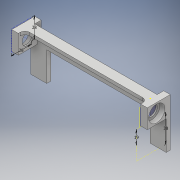
# Autodesk Inventor part: rearAxelHolder 9-19
Saved by Autodesk Inventor 2018 (Build 220112000, 112)
## iProperties
Created: 2019-09-19
Part Number: rearAxelHolder 9-19
Material: Generic
Document SubType Name: Modeling
Designer: Aditya Kendre
Density: 1 g/cm^3
Appearance: Default
Author: Aditya Kendre
Autodesk Inventor part; units mm, degrees
ref_plane "YZ Plane" through (0, 0, 0) normal (1, 0, 0) x (0, 1, 0)
ref_plane "XZ Plane" through (0, 0, 0) normal (0, 1, 0) x (-1, 0, 0)
ref_plane "XY Plane" through (0, 0, 0) normal (0, 0, 1) x (1, 0, 0)
sketch "Sketch1" plane through (0, 0, 0) normal (1, 0, 0) x (0, 1, 0)
  circle A0 centre (0, 0) radius 11.25
  line L0 (-11.25, 11.25) -> (11.25, 11.25) construction
  line L1 (11.25, 11.25) -> (11.25, -11.25) construction
  line L2 (11.25, -11.25) -> (-11.25, -11.25) construction
  line L3 (-11.25, -11.25) -> (-11.25, 11.25) construction
  line L4 (-11.25, 11.25) -> (11.25, -11.25) construction
  line L5 (11.25, 11.25) -> (-11.25, -11.25) construction
  line L6 (11.25, 11.25) -> (14.25, 11.25) construction
  line L7 (14.25, 11.25) -> (14.25, -11.25) construction
  line L8 (14.25, -11.25) -> (11.25, -11.25) construction
  line L9 (11.25, -11.25) -> (11.25, 11.25) construction
  line L10 (14.25, -11.25) -> (-11.25, -11.25) construction
  line L11 (-11.25, -11.25) -> (-11.25, -14.25) construction
  line L12 (-11.25, -14.25) -> (14.25, -14.25) construction
  line L13 (14.25, -14.25) -> (14.25, -11.25) construction
  line L14 (-13, 13) -> (13, 13)
  line L15 (13, 13) -> (13, -13)
  line L16 (13, -13) -> (-13, -13)
  line L17 (-13, -13) -> (-13, 13)
  line L18 (-13, 13) -> (13, -13) construction
  line L19 (13, 13) -> (-13, -13) construction
  dimension "d0" = 22.5
  dimension "d1" = 3
  dimension "d2" = 3
  dimension "d3" = 26
  dimension "d4" = 26
  constraints: 40 end point, 8 parallel, 4 horizontal, 4 midpoint, 4 perpendicular, 1 centre point, 1 coincident
  measures "d0" diameter of A0
  measures "d1" distance of L7.end L8.end
  measures "d2" distance of L11.end L10.end
  measures "d3" distance of L15.end L16.end
  measures "d4" distance of L14.end L15.end
extrude "Extrusion1" add sketch "Sketch1" along normal blind 9
sketch "Sketch2" plane through (0, 0, 0) normal (-1, 0, 0) x (0, 0, 1)
  circle A0 centre (0, 0) radius 7.75
  circle A1 centre (0, 0) radius 11.25
  dimension "d7" = 15.5
  constraints: 2 centre point, 2 coincident
  measures "d7" diameter of A0
extrude "Extrusion2" add sketch "Sketch2" against normal blind 2
sketch "Sketch3" plane through (0, 0, 0) normal (-1, 0, 0) x (0, 0, 1)
  line L0 (13, 13) -> (-13, 13) projected
  line L1 (13, 13) -> (8.75, 13)
  line L2 (8.75, 13) -> (8.75, -13)
  line L3 (8.75, -13) -> (13, -13)
  line L4 (13, -13) -> (13, 13)
  point P0 (0, 0)
  dimension "d10" = 4.25
  dimension "d11" = 26
  constraints: 8 end point, 2 parallel, 1 horizontal, 1 perpendicular
  measures "d10" distance of L3.end L2.end
  measures "d11" distance of L2.end L1.end
extrude "Extrusion3" add sketch "Sketch3" along normal blind 168
sketch "Sketch4" plane through (-168, 0, 0) normal (-1, 0, 0) x (0, 0, 1)
  line L0 (13, 13) -> (13, -13) projected
  line L1 (-13, -13) -> (-13, 13) projected
  line L2 (13, -13) -> (-13, -13)
  line L3 (-13, -13) -> (-13, 13)
  line L4 (-13, 13) -> (13, 13)
  line L5 (13, 13) -> (13, -13)
  circle A0 centre (0, 0) radius 7.75
  circle A1 centre (0, 0) radius 11.25
  constraints: 8 end point, 2 centre point, 2 coincident, 2 parallel, 1 horizontal, 1 perpendicular
extrude "Extrusion4" add sketch "Sketch4" along normal blind 9 contours L0 L2 L1 L4
sketch "Sketch5" plane through (-168, 0, 0) normal (1, 0, 0) x (0, 0, -1)
  circle A0 centre (0, 0) radius 7.75
  circle A1 centre (0, 0) radius 11.25
  constraints: 2 centre point, 2 coincident
extrude "Extrusion5" add sketch "Sketch5" against normal blind 2
sketch "Sketch6" plane through (0, 13, -13) normal (0, 1, 0) x (1, 0, 0)
  line L0 (9, -26) -> (9, 0) projected
  line L1 (-177, -26) -> (-177, 0) projected
  line L2 (9, 0) -> (-177, 0)
  line L3 (-177, 0) -> (-177, -26)
  line L4 (-177, -26) -> (9, -26)
  line L5 (9, -26) -> (9, 0)
  point P0 (0, -13)
  constraints: 8 end point, 2 parallel, 1 horizontal, 1 perpendicular
extrude "Extrusion6" add sketch "Sketch6" along normal blind 5.5
ref_plane "Work Plane1" through (0, 0, 0) normal (-1, 0, 0) x (0, 0, 1)
sketch "Sketch7" plane through (0, 0, 0) normal (-1, 0, 0) x (0, 0, 1)
  line L0 (13, -13) -> (13, 18.5) projected
  line L1 (13, 18.5) -> (3.75, 18.5)
  line L2 (3.75, 18.5) -> (3.75, 9.5)
  line L3 (3.75, 9.5) -> (13, 9.5)
  line L4 (13, 9.5) -> (13, 18.5)
  point P0 (0, 0)
  dimension "d21" = 9.25
  dimension "d22" = 9
  constraints: 8 end point, 2 parallel, 1 horizontal, 1 perpendicular
  measures "d21" distance of L3.end L2.end
  measures "d22" distance of L2.end L1.end
extrude "Extrusion7" cut sketch "Sketch7" along normal blind 168
sketch "Sketch8" plane through (0, 0, 0) normal (-1, 0, 0) x (0, 0, 1)
  point P0 (0, 0)
sketch "Sketch9" plane through (-177, -13, 13) normal (0, 0, 1) x (1, 0, 0)
  point P0 (177, 13)
sketch "Sketch10" plane through (-177, -13, 13) normal (0, 0, 1) x (1, 0, 0)
  line L0 (0, 0) -> (0, 31.5) construction
  line L1 (9, 0) -> (0, 0) construction
  line L2 (0, 31.5) -> (9, 31.5) construction
  line L3 (9, 31.5) -> (9, 0) construction
  line L4 (9, 0) -> (0, 0) construction
  line L5 (0, 0) -> (0, 31.5) construction
  line L6 (186, 31.5) -> (0, 31.5) construction
  line L7 (0, 0) -> (186, 0) construction
  line L8 (186, 31.5) -> (177, 31.5) construction
  line L9 (177, 31.5) -> (177, 0) construction
  line L10 (177, 0) -> (186, 0) construction
  line L11 (186, 0) -> (186, 31.5) construction
  line L12 (9, 22.5) -> (9, 0) projected
  line L13 (177, 0) -> (177, 22.5) projected
  line L14 (9, 0) -> (177, 0)
  line L15 (177, 0) -> (177, 9)
  line L16 (177, 9) -> (9, 9)
  line L17 (9, 9) -> (9, 0)
  point P0 (177, 13)
  dimension "d25" = 9
  constraints: 24 end point, 6 parallel, 3 horizontal, 3 perpendicular, 2 point on line
  measures "d25" distance of L15.end L14.end
extrude "Extrusion8" cut sketch "Sketch10" against normal blind 5
fillet "Fillet1" radius 6.5 2 edges at (0, -4, 10.875) (-168, -4, 10.875)
sketch "Sketch11" plane through (9, -13, -13) normal (0, 0, -1) x (-1, 0, 0)
  point P0 (9, 13)
sketch "Sketch12" plane through (9, -13, -13) normal (0, 0, -1) x (-1, 0, 0)
  line L0 (0, 31.5) -> (186, 31.5) construction
  line L1 (9, 26) -> (177, 26) construction
  line L2 (0, 31.5) -> (22, 31.5) construction
  line L3 (22, 31.5) -> (22, 26) construction
  line L4 (22, 26) -> (0, 26) construction
  line L5 (0, 26) -> (0, 31.5) construction
  line L6 (17.1, 27.15) -> (4.9, 27.15) construction
  line L7 (4.9, 27.15) -> (4.9, 30.35) construction
  line L8 (4.9, 30.35) -> (17.1, 30.35) construction
  line L9 (17.1, 30.35) -> (17.1, 27.15) construction
  line L10 (17.1, 27.15) -> (4.9, 30.35) construction
  line L11 (4.9, 27.15) -> (17.1, 30.35) construction
  line L12 (17.1, 27.15) -> (4.9, 27.15)
  line L13 (4.9, 27.15) -> (4.9, 30.35)
  line L14 (4.9, 30.35) -> (17.1, 30.35)
  line L15 (17.1, 30.35) -> (17.1, 27.15)
  line L16 (17.1, 27.15) -> (4.9, 30.35) construction
  line L17 (4.9, 27.15) -> (17.1, 30.35) construction
  line L18 (186, 0) -> (186, 31.5) construction
  line L19 (186, 31.5) -> (164, 31.5) construction
  line L20 (164, 31.5) -> (164, 26) construction
  line L21 (164, 26) -> (186, 26) construction
  line L22 (186, 26) -> (186, 31.5) construction
  line L23 (181.1, 27.15) -> (168.9, 27.15)
  line L24 (168.9, 27.15) -> (168.9, 30.35)
  line L25 (168.9, 30.35) -> (181.1, 30.35)
  line L26 (181.1, 30.35) -> (181.1, 27.15)
  line L27 (181.1, 27.15) -> (168.9, 30.35) construction
  line L28 (168.9, 27.15) -> (181.1, 30.35) construction
  line L29 (22, 26) -> (0, 26)
  line L30 (0, 26) -> (0, 31.5)
  line L31 (0, 31.5) -> (22, 31.5)
  line L32 (22, 31.5) -> (22, 26)
  line L33 (164, 26) -> (186, 26)
  line L34 (186, 26) -> (186, 31.5)
  line L35 (186, 31.5) -> (164, 31.5)
  line L36 (164, 31.5) -> (164, 26)
  point P0 (9, 13)
  point P1 (11, 28.75)
  point P2 (175, 28.75)
  dimension "d29" = 22
  dimension "d30" = 12.2
  dimension "d31" = 3.2
  dimension "d32" = 22
  dimension "d33" = 12.2
  dimension "d34" = 3.2
  constraints: 68 end point, 14 parallel, 7 horizontal, 7 perpendicular, 6 midpoint, 2 point on line
  measures "d29" distance of L3.end L4.end
  measures "d30" distance of L7.end L8.end
  measures "d31" distance of L6.end L7.end
  measures "d32" distance of L21.end L20.end
  measures "d33" distance of L24.end L25.end
  measures "d34" distance of L23.end L24.end
extrude "Extrusion9" add sketch "Sketch12" along normal blind 40
sketch "Sketch13" plane through (4.1, 17.35, -13) normal (0, 0, -1) x (-1, 0, 0)
  line L0 (0, 0) -> (12.2, 0) projected
  line L1 (0, -3.2) -> (12.2, -3.2) projected
  line L2 (0, 0) -> (12.2, 0)
  line L3 (12.2, 0) -> (12.2, -3.2)
  line L4 (12.2, -3.2) -> (0, -3.2)
  line L5 (0, -3.2) -> (0, 0)
  line L6 (176.2, 0) -> (164, 0) projected
  line L7 (164, -3.2) -> (176.2, -3.2) projected
  line L8 (164, 0) -> (176.2, 0)
  line L9 (176.2, 0) -> (176.2, -3.2)
  line L10 (176.2, -3.2) -> (164, -3.2)
  line L11 (164, -3.2) -> (164, 0)
  point P0 (4.1, -17.35)
  constraints: 16 end point, 4 parallel, 2 horizontal, 2 perpendicular
extrude "Extrusion10" cut sketch "Sketch13" against normal blind 15
sketch "Sketch14" plane through (-177, 0, 0) normal (-1, 0, 0) x (0, 0, 1)
  line L0 (14, -14) -> (-14, -14) construction
  line L1 (-14, -14) -> (-14, 14) construction
  line L2 (-14, 14) -> (14, 14) construction
  line L3 (14, 14) -> (14, -14) construction
  line L4 (14, -14) -> (-14, 14) construction
  line L5 (-14, -14) -> (14, 14) construction
  point P0 (0, 0)
  dimension "d39" = 28
  dimension "d40" = 28
  constraints: 12 end point, 2 midpoint, 2 parallel, 1 horizontal, 1 perpendicular
  measures "d39" distance of L1.end L2.end
  measures "d40" distance of L0.end L1.end
sketch "Sketch15" plane through (0, 0, 0) normal (-1, 0, 0) x (0, 0, 1)
  line L0 (-33, -19) -> (-14, -19) construction
  line L1 (-14, -19) -> (-14, 0) construction
  line L2 (-33, 19) -> (-14, 19) construction
  line L3 (-14, -19) -> (-52, -19) construction
  line L4 (-52, -19) -> (-52, 19) construction
  line L5 (-52, 19) -> (-14, 19) construction
  point P0 (0, 0)
  dimension "d41" = 19
  dimension "d45" = 38
  constraints: 12 end point, 1 horizontal, 1 parallel, 1 perpendicular, 1 point on line
  measures "d41" distance of L0.end L0.start
  measures "d45" distance of L4.end L5.end
body "Solid1"
